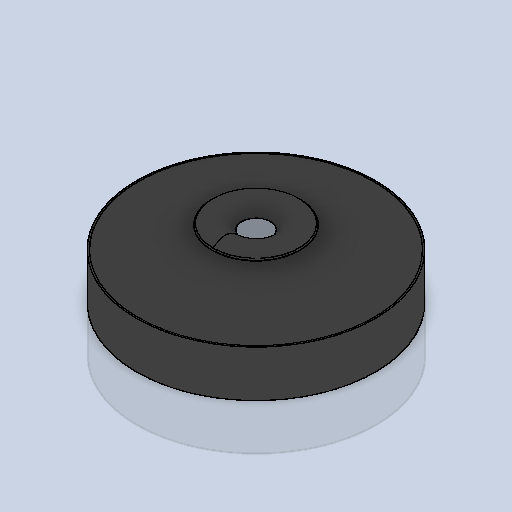
# Autodesk Inventor part: rubber_sleeve
Saved by Autodesk Inventor 2026.1 (Build 301233000, 233)
## iProperties
Created: 2025-09-05
Part Number: rubber_sleeve
Material: Rubber
Document SubType Name: Modeling
Designer: baseb
Density: 0.93 g/cm^3
Appearance: Rubber - Black
Author: baseb
Autodesk Inventor part; units mm, degrees
ref_plane "YZ Plane" through (0, 0, 0) normal (1, 0, 0) x (0, 1, 0)
ref_plane "XZ Plane" through (0, 0, 0) normal (0, 1, 0) x (-1, 0, 0)
ref_plane "XY Plane" through (0, 0, 0) normal (0, 0, 1) x (1, 0, 0)
sketch "Sketch1" plane through (0, 0, 0) normal (1, 0, 0) x (0, 1, 0)
  line L0 (16.3991, -98.278) -> (51.3241, -72.878) construction
  line L1 (51.3241, -72.878) -> (51.3241, -74.402) construction
  line L2 (51.3241, -74.402) -> (16.3991, -99.802) construction
  line L3 (0, -113.538) -> (16.3991, -113.538)
  line L4 (0, 0.762) -> (0, -0.762)
  line L5 (0, 0.762) -> (16.3991, -98.278)
  line L6 (0, -0.762) -> (16.3991, -99.802)
  line L7 (16.3991, -99.802) -> (16.3991, -98.278)
  line L8 (16.3991, -98.278) -> (33.1367, -86.1052) construction
  line L9 (33.1367, -86.1052) -> (19.6348, -72.4523) construction
  spline S0 degree 2 poles (16.3991, -98.278) (33.1367, -86.1052) (19.6348, -72.4523) knots 1 1 1 2 2 2
  line L10 (19.6348, -72.4523) -> (20.7184, -71.3806)
  line L11 (16.3991, -99.802) -> (33.8616, -87.102) construction
  line L12 (33.8616, -87.102) -> (21.7781, -72.4523) construction
  spline S1 degree 2 poles (16.3991, -99.802) (33.8616, -87.102) (21.7781, -72.4523) knots 1 1 1 2 2 2
  line L13 (21.7781, -72.4523) -> (20.7184, -71.3806)
  line L14 (0, 0.762) -> (-44.45, 0.762)
  line L15 (-44.45, 0.762) -> (-44.45, -0.762)
  line L16 (-44.45, -0.762) -> (0, -0.762)
  line L17 (0, -0.762) -> (0, 0.762)
  point P0 (0, 0)
  dimension "d5" = 1.524
  dimension "d8" = 34.925
  dimension "d26" = 1.524
  dimension "d27" = 1.524
  dimension "d28" = 1.524
  dimension "d30" = 44.45
  dimension "d31" = 1.524
  dimension "d32" = 114.3
  constraints: 28 end point, 3 parallel, 2 horizontal, 2 midpoint, 2 perpendicular, 2 point on line, 2 vertical, 6 other
  measures "d5" distance of L0.end L1.end
  measures "d8" horizontal distance of L2.end L0.end
  measures "d26" distance of L4.start L4.end
  measures "d27" distance of L6.end L5.end
  measures "d28" distance of L9.end L10.end
  measures "d30" distance of L15.end L16.end
  measures "d31" distance of L14.end L15.end
  measures "d32" distance from line of L4.start L3
revolve "Revolution2" add sketch "Sketch1" angle 360 about axis through (0, 0, -113.538) along (0, 1, 0)
body "Solid2"
